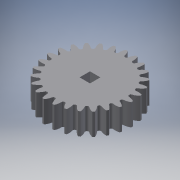
# Autodesk Inventor part: gear 2 shaft
Saved by Autodesk Inventor 2017 (Build 210142000, 142)
## iProperties
Created: 2018-04-17
Part Number: gear 2 shaft
Material: Generic
Document SubType Name: Modeling
Designer: RKL
Density: 1 g/cm^3
Appearance: Default
Author: RKL
Autodesk Inventor part; units mm, degrees
ref_plane "YZ Plane" through (0, 0, 0) normal (1, 0, 0) x (0, 1, 0)
ref_plane "XZ Plane" through (0, 0, 0) normal (0, 1, 0) x (-1, 0, 0)
ref_plane "XY Plane" through (0, 0, 0) normal (0, 0, 1) x (1, 0, 0)
sketch "Sketch1" plane through (0, 0, 0) normal (0, 0, 1) x (1, 0, 0)
  spline S0 degree 3 poles (-3.7631, 38.3127) (-3.5822, 38.0454) (-3.2202, 37.5109) (-2.7372, 36.6712) (-2.3047, 35.8041) (-1.9449, 34.9056) (-1.7049, 34.1314) (-1.6187, 33.4912) (-1.493, 33.0221) (-1.3119, 32.6569) (-1.1068, 32.4058) (-0.9204, 32.2507) (-0.7164, 32.1178) (-0.4042, 32.0239) (0, 32.0176) (0.4042, 32.0239) (0.7164, 32.1178) (0.9204, 32.2507) (1.1068, 32.4058) (1.3119, 32.6569) (1.493, 33.0221) (1.6187, 33.4912) (1.7049, 34.1314) (1.9449, 34.9056) (2.3047, 35.8041) (2.7372, 36.6712) (3.2202, 37.5109) (3.5822, 38.0454) (3.7631, 38.3127) knots 0 0 0 0 0.096801 0.193601 0.290398 0.387185 0.483936 0.532341 0.580735 0.629067 0.653298 0.677436 0.701607 0.7258 0.774017 0.822235 0.846427 0.870598 0.894737 0.918967 0.9673 1.015693 1.064099 1.16085 1.257636 1.354433 1.451234 1.548035 1.548035 1.548035 1.548035
  circle A0 centre (0, 0) radius 32.0201 construction
  circle A1 centre (0, 0) radius 33.594 construction
  circle A2 centre (0, 0) radius 35.75 construction
  circle A3 centre (0, 0) radius 38.4971
  point P0 (-3.2302, 37.5046)
  point P1 (-2.7456, 36.6666)
  point P2 (-2.3168, 35.7988)
  point P3 (-1.9568, 34.9004)
  point P4 (-1.6922, 33.9698)
  point P5 (-1.6085, 33.493)
  point P6 (-1.4777, 33.0271)
  point P7 (-1.2557, 32.5977)
  point P8 (-1.1012, 32.4111)
  point P9 (-0.9176, 32.2544)
  point P10 (-0.7114, 32.1282)
  point P11 (-0.4809, 32.0547)
  point P12 (0, 32.0201)
  point P13 (0.4809, 32.0547)
  point P14 (0.7114, 32.1282)
  point P15 (0.9176, 32.2544)
  point P16 (1.1012, 32.4111)
  point P17 (1.2557, 32.5977)
  point P18 (1.4777, 33.0271)
  point P19 (1.6085, 33.493)
  point P20 (1.6922, 33.9698)
  point P21 (1.9568, 34.9004)
  point P22 (2.3168, 35.7988)
  point P23 (2.7456, 36.6666)
  point P24 (3.2302, 37.5046)
  constraints: 4 centre point, 2 point on circle, 59 other
extrude "Extrusion1" add sketch "Sketch1" against normal blind 20
extrude "Extrusion2" cut sketch "Sketch1" against normal through all contours A3 S0 picked at (-0.4594, 36.8)
pattern_circular "Circular Pattern1" count 26 over 360 about axis through (0, 0, 0) along (0, 0, -1) of "Extrusion2"
sketch "Sketch2" plane through (0, 0, 0) normal (0, 0, 1) x (1, 0, 0)
  line L0 (4.7625, -4.7625) -> (-4.7625, -4.7625)
  line L1 (-4.7625, -4.7625) -> (-4.7625, 4.7625)
  line L2 (-4.7625, 4.7625) -> (4.7625, 4.7625)
  line L3 (4.7625, 4.7625) -> (4.7625, -4.7625)
  line L4 (4.7625, -4.7625) -> (-4.7625, 4.7625) construction
  line L5 (-4.7625, -4.7625) -> (4.7625, 4.7625) construction
  point P0 (0, 0)
  dimension "d7" = 9.525
  constraints: 12 end point, 2 midpoint, 2 parallel, 2 perpendicular, 1 horizontal
  measures "d7" distance of L0.end L1.end
extrude "Extrusion3" cut sketch "Sketch2" against normal through all
equation "\"d0\" = FaceWidth"
equation "\"Module\" = 2.75"
equation "\"PressureAngle\" = 20deg"
equation "\"UnitProfileClearance\" = 0.25"
equation "\"UnitRoundRadius\" = 0.35"
equation "\"HeadDiameter\" = 76.99415"
equation "\"RootDiameter\" = 64.04024"
equation "\"BaseDiameter\" = 67.18802"
equation "\"PitchDiameter\" = 71.5"
equation "\"FaceWidth\" = 20"
equation "\"HelixAngle\" = 0"
equation "\"UnitCorrection\" = 0"
equation "\"UnitAddendumModification\" = 0.001064"
equation "\"CircularPitch\" = 8.63938"
equation "\"UnitBacklashShift\" = -0.10632"
equation "\"TotalToolShift\" = -0.29238"
equation "\"IsInternal\" = 0"
body "Solid1"
